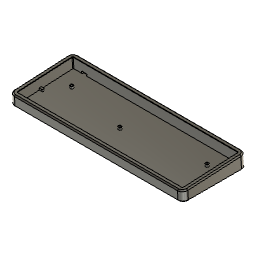
MFR60 (Autodesk Fusion 360 design; units mm, degrees)
Autodesk Fusion 360 part; units mm, degrees
note: some values were not read from the file. Set by a fixed rule: which sketch regions a step uses.
sketch "PCB Plane" plane through (0, 0, 0) normal (0, 0, 1) x (1, 0, 0)
  line L0 (0, 0) -> (285.75, 0) construction
  line L1 (285.75, 0) -> (285.75, 95.25) construction
  line L2 (285.75, 95.25) -> (0, 95.25) construction
  line L3 (0, 95.25) -> (0, 0) construction
  line L4 (-0.5, -0.5) -> (286.25, -0.5)
  line L5 (286.25, -0.5) -> (286.25, 95.75)
  line L6 (286.25, 95.75) -> (-0.5, 95.75)
  line L7 (-0.5, 95.75) -> (-0.5, -0.5)
  line L8 (-7.5, 102.75) -> (-7.5, -7.5)
  line L9 (-7.5, -7.5) -> (293.25, -7.5)
  line L10 (293.25, -7.5) -> (293.25, 102.75)
  line L11 (293.25, 102.75) -> (-7.5, 102.75)
  dimension "d1" = 285.75
  dimension "d2" = 95.25
  dimension "d3" = 0.5
  dimension "d4" = 7.5
  constraint horizontal L0
  constraint vertical L1
  constraint horizontal L2
  constraint vertical L3
  constraint coincident L0.start L3.end
  measures "d1" distance of L0.start L0.end
  measures "d2" distance of L0.start L2.end
ref_plane "WorkPlane1" through (142.875, 47.625, -3.46) normal (0, 0, 1) x (1, 0, 0)
ref_plane "WorkPlane2" through (142.875, 47.625, 14.6) normal (0, 0, 1) x (1, 0, 0)
extrude "Extrude1" add sketch "PCB Plane" along normal up to surface (14.6 mm away) and the other way up to surface (3.46 mm away)
sketch "Angle Sketch" plane through (293.25, 0, 0) normal (1, 0, 0) x (0, 1, 0)
  line L0 (102.75, 14.6) -> (-7.5, 14.6)
  line L1 (-7.5, 14.6) -> (-7.5, -3.46)
  line L2 (-7.5, -3.46) -> (102.75, -3.46)
  line L3 (102.75, -3.46) -> (102.75, 14.6)
  line L4 (-7.5, 14.6) -> (-7.5, -3.6755)
  line L5 (-7.5, -3.6755) -> (92.363, -8.9091)
  line L6 (-7.5, -3.6755) -> (92.5, -3.6755) construction
  dimension "d11" = 18.2755
  dimension "d12" = 100
  dimension "d13" = 3
  constraint coincident L0.end L1.start
  constraint perpendicular L0 L4
  constraint horizontal L6
  measures "d11" distance of L0.end L4.end
  measures "d12" distance of L4.end L5.end
  measures "d13" angle of L5 L6
ref_plane "WorkPlane3" through (293.25, 42.4315, -6.2923) normal (0, -0.052336, -0.99863) x (0, 0.99863, -0.052336)
sketch "Interior Base Plane" plane through (0, 0, -3.46) normal (0, 0, -1) x (1, 0, 0)
  line L0 (286.25, -95.75) -> (-0.5, -95.75)
  line L1 (-0.5, -95.75) -> (-0.5, 0.5)
  line L2 (-0.5, 0.5) -> (286.25, 0.5)
  line L3 (286.25, 0.5) -> (286.25, -95.75)
  line L4 (-7.5, 7.5) -> (-7.5, -102.75)
  line L5 (-7.5, -102.75) -> (293.25, -102.75)
  line L6 (293.25, -102.75) -> (293.25, 7.5)
  line L7 (293.25, 7.5) -> (-7.5, 7.5)
  line L8 (-7.5, 7.5) -> (293.25, 7.5)
  line L9 (293.25, 7.5) -> (293.25, -102.75)
  line L10 (293.25, -102.75) -> (-7.5, -102.75)
  line L11 (-7.5, -102.75) -> (-7.5, 7.5)
  constraint horizontal L8
  constraint vertical L9
  constraint horizontal L10
  constraint vertical L11
  constraint coincident L5.end L6.start
  constraint coincident L4.start L7.end
extrude "Extrude2" add sketch "Interior Base Plane" along normal up to surface contours L0 L1 L2 L3 | L4 L5 L6 L7 L8 L9 L10 L11 end surface through (293.25, 42.4315, -6.2923) normal (0, -0.052336, -0.99863) offset 0
fillet "Fillet1" radius 9 1 edges at (293.25, -7.5, 5.4623)
fillet "Fillet2" radius 9 1 edges at (293.25, 102.75, 2.5733)
fillet "Fillet3" radius 9 1 edges at (-7.5, 102.75, 2.5733)
fillet "Fillet4" radius 9 1 edges at (-7.5, -7.5, 5.4623)
fillet "Fillet5" radius 1 1 edges at (286.25, 95.75, 5.57)
fillet "Fillet6" radius 1 1 edges at (-0.5, 95.75, 5.57)
fillet "Fillet7" radius 1 1 edges at (286.25, -0.5, 5.57)
fillet "Fillet8" radius 1 1 edges at (-0.5, -0.5, 5.57)
chamfer "Chamfer1" distance 2 angle 45 8 edges at (-7.5, 47.625, 14.6) (-4.864, 100.114, 14.6) (142.875, 102.75, 14.6) (290.614, 100.114, 14.6) (293.25, 47.625, 14.6) (290.614, -4.864, 14.6) (142.875, -7.5, 14.6) (-4.864, -4.864, 14.6)
chamfer "Chamfer2" distance 2 angle 45 8 edges at (-7.5, 47.625, -6.5645) (-4.864, -4.864, -3.8136) (142.875, -7.5, -3.6755) (290.614, -4.864, -3.8136) (293.25, 47.625, -6.5645) (290.614, 100.114, -9.3153) (142.875, 102.75, -9.4535) (-4.864, 100.114, -9.3153)
chamfer "Chamfer3" distance 0.5 angle 45 4 edges at (142.875, 95.75, 14.6) (-0.5, 47.625, 14.6) (142.875, -0.5, 14.6) (286.25, 47.625, 14.6)
extrude "Extrude3" add 1 faces at (190, 65.3342, -7.4926) along direction (0, 0.052336, 0.99863) blind 1
ref_plane "WorkPlane4" through (142.875, 47.625, 0) normal (0, 0, 1) x (1, 0, 0)
sketch "USB C Hole Internal" plane through (0, 95.75, 0) normal (0, -1, 0) x (1, 0, 0)
  line L0 (285.25, 14.1) -> (0.5, 14.1)
  line L1 (0.5, -3.46) -> (285.25, -3.46)
  line L2 (15.4, -3.46) -> (21.75, -3.46)
  line L3 (23.3, -1.91) -> (23.3, -1.35)
  line L4 (21.75, 0.2) -> (15.4, 0.2)
  line L5 (13.85, -1.35) -> (13.85, -1.91)
  arc A0 (15.4, 0.2) -> (13.85, -1.35) centre (15.4, -1.35) ccw
  arc A1 (23.3, -1.35) -> (21.75, 0.2) centre (21.75, -1.35) ccw
  arc A2 (21.75, -3.46) -> (23.3, -1.91) centre (21.75, -1.91) ccw
  arc A3 (13.85, -1.91) -> (15.4, -3.46) centre (15.4, -1.91) ccw
  line L6 (0.5, 14.1) -> (0.5, -3.46)
  line L7 (285.25, -3.46) -> (285.25, 14.1)
  line L8 (285.25, -0.2545) -> (285.75, -0.2545)
  line L9 (18.575, 0.2) -> (18.575, -3.46) construction
  line L10 (285.75, -0.2545) -> (285.375, -0.2545)
  dimension "d36" = 1.55
  dimension "d82" = 0.5
  dimension "d83" = 4.725
  dimension "d89" = 3.66
  dimension "d90" = 3.66
  dimension "d132" = 0.375
  dimension "d133" = 266.8
  constraint horizontal L2
  constraint vertical L3
  constraint horizontal L4
  constraint vertical L5
  constraint tangent L5 A0
  constraint tangent L4 A0
  constraint tangent L4 A1
  constraint tangent L3 A1
  constraint equal A0 A1
  constraint tangent L2 A2
  constraint tangent L3 A2
  constraint equal A0 A2
  constraint tangent L2 A3
  constraint tangent L5 A3
  constraint equal A0 A3
  constraint coincident L7 L8.start
  constraint perpendicular L7 L8
  constraint midpoint L4 L9.start
  constraint midpoint L2 L9.end
  constraint perpendicular L7 L10
  measures "d36" radius of A0
  measures "d82" distance of L8.start L8.end
  measures "d83" distance of L5 L9
  measures "d89" distance of L2 L4
  measures "d90" distance of L1 L4
  measures "d132" distance of L8.end L10.end
  measures "d133" distance of L9 L10.end
extrude "Extrude4" cut sketch "USB C Hole Internal" against normal through all contours L1 L2 L3 L4 L5 A0 A1 A2 A3
sketch "USB C Hole External" plane through (0, 102.75, 0) normal (0, 1, 0) x (-1, 0, 0)
  line L0 (-21.75, 0.2) -> (-15.4, 0.2)
  arc A0 (-13.85, -1.35) -> (-15.4, 0.2) centre (-15.4, -1.35) ccw
  line L1 (-13.85, -1.35) -> (-13.85, -1.91)
  arc A1 (-15.4, -3.46) -> (-13.85, -1.91) centre (-15.4, -1.91) ccw
  line L2 (-15.4, -3.46) -> (-21.75, -3.46)
  arc A2 (-23.3, -1.91) -> (-21.75, -3.46) centre (-21.75, -1.91) ccw
  line L3 (-23.3, -1.91) -> (-23.3, -1.35)
  arc A3 (-21.75, 0.2) -> (-23.3, -1.35) centre (-21.75, -1.35) ccw
  line L4 (-284.25, -7.4535) -> (-1.5, -7.4535)
  line L5 (-1.5, -7.4535) -> (-1.5, 12.6)
  line L6 (-1.5, 12.6) -> (-284.25, 12.6)
  line L7 (-284.25, 12.6) -> (-284.25, -7.4535)
  line L8 (-13.85, -1.63) -> (-23.3, -1.63) construction
  line L9 (-18.575, 0.2) -> (-18.575, -3.46) construction
  line L10 (-19.075, 2.45) -> (-19.075, -5.71) construction
  line L11 (-190.8318, -1.63) -> (-176.8818, -1.63) construction
  line L12 (-21.75, 2.45) -> (-15.4, 2.45)
  line L13 (-11.6, -1.35) -> (-11.6, -1.91)
  line L14 (-15.4, -5.71) -> (-21.75, -5.71)
  line L15 (-25.55, -1.91) -> (-25.55, -1.35)
  arc A4 (-25.55, -1.91) -> (-21.75, -5.71) centre (-21.75, -1.91) ccw
  arc A5 (-21.75, 2.45) -> (-25.55, -1.35) centre (-21.75, -1.35) ccw
  arc A6 (-11.6, -1.35) -> (-15.4, 2.45) centre (-15.4, -1.35) ccw
  arc A7 (-15.4, -5.71) -> (-11.6, -1.91) centre (-15.4, -1.91) ccw
  dimension "d39" = 8.16
  dimension "d40" = 4.08
  dimension "d42" = 13.95
  dimension "d43" = 3.8
  dimension "d85" = 13.95
  dimension "d86" = 8.16
  dimension "d87" = 6.975
  dimension "d88" = 4.08
  constraint midpoint L1 L8.start
  constraint midpoint L3 L8.end
  constraint midpoint L0 L9.start
  constraint midpoint L2 L9.end
  constraint perpendicular L2 L10
  constraint perpendicular L10 L11
  constraint horizontal L12
  constraint vertical L13
  constraint horizontal L14
  constraint vertical L15
  constraint tangent L14 A4
  constraint tangent L15 A4
  constraint tangent L15 A5
  constraint tangent L12 A5
  constraint equal A4 A5
  constraint tangent L12 A6
  constraint tangent L13 A6
  constraint equal A4 A6
  constraint tangent L13 A7
  constraint tangent L14 A7
  constraint equal A4 A7
  measures "d39" distance of L10.start L10.end
  measures "d40" distance of L8 L10.start
  measures "d42" distance of L11.start L11.end
  measures "d43" radius of A4
  measures "d85" distance of L13 L15
  measures "d86" distance of L12 L14
  measures "d87" distance of L9 L15
  measures "d88" distance of L8.end L14
extrude "Extrude5" cut sketch "USB C Hole External" against normal blind 4.5025 contours L12 L13 L14 L15 A4 A5 A6 A7
chamfer "Chamfer4" distance 0.25 angle 45 8 edges at (24.437, 102.75, -4.597) (25.55, 102.75, -1.63) (24.437, 102.75, 1.337) (18.575, 102.75, 2.45) (12.713, 102.75, 1.337) (11.6, 102.75, -1.63) (12.713, 102.75, -4.597) (18.575, 102.75, -5.71)
sketch "Hole Tops" plane through (0, 0, 0) normal (0, 0, 1) x (1, 0, 0)
  line L0 (0, 0) -> (195.2625, 0) construction
  line L1 (195.2625, 0) -> (195.2625, 76.2) construction
  line L2 (195.2625, 76.2) -> (0, 76.2) construction
  line L3 (0, 76.2) -> (0, 0) construction
  line L4 (195.2625, 76.2) -> (195.2625, 57.15) construction
  line L5 (195.2625, 57.15) -> (193.1449, 57.15) construction
  circle A0 centre (157.1625, 57.15) radius 2.75
  circle A1 centre (38.1, 57.15) radius 2.75
  circle A2 centre (38.1, 19.05) radius 2.75
  circle A3 centre (157.1625, 19.05) radius 2.75
  dimension "d47" = 195.2625
  dimension "d48" = 76.2
  dimension "d51" = 19.05
  dimension "d52" = 38.1
  dimension "d53" = 19.05
  dimension "d54" = 38.1
  dimension "d55" = 38.1
  dimension "d56" = 19.05
  dimension "d57" = 38.1
  dimension "d58" = 19.05
  dimension "d59" = 5.5
  constraint horizontal L0
  constraint vertical L1
  constraint horizontal L2
  constraint vertical L3
  constraint coincident L0.start L3.end
  constraint perpendicular L2 L4
  constraint perpendicular L1 L5
  constraint equal A0 A1
  constraint equal A0 A3
  constraint equal A1 A2
  measures "d47" distance of L0.start L0.end
  measures "d48" distance of L0.start L2.end
  measures "d51" distance of L2 A0.centre
  measures "d52" distance of L1 A0.centre
  measures "d53" distance of L0 A3.centre
  measures "d54" distance of L1 A3.centre
  measures "d55" distance of L3 A2.centre
  measures "d56" distance of L0 A2.centre
  measures "d57" distance of L3 A1.centre
  measures "d58" distance of L2 A1.centre
  measures "d59" diameter of A1
sketch "Screwpost Positions" plane through (0, 0, -3.46) normal (0, 0, 1) x (-1, 0, 0)
  line L0 (0.5, -7.4953) -> (-286.25, -7.4953)
  line L1 (-286.25, -7.4953) -> (-286.25, -94.75)
  line L2 (-15.4, -95.75) -> (-0.5, -95.75)
  line L3 (0.5, -94.75) -> (0.5, -7.4953)
  line L4 (-21.75, -98.2475) -> (-15.4, -98.2475)
  line L5 (-15.4, -98.2475) -> (-15.4, -95.75)
  arc A0 (-0.5, -95.75) -> (0.5, -94.75) centre (-0.5, -94.75) ccw
  arc A1 (-286.25, -94.75) -> (-285.25, -95.75) centre (-285.25, -94.75) ccw
  line L6 (-285.25, -95.75) -> (-21.75, -95.75)
  line L7 (-21.75, -95.75) -> (-21.75, -98.2475)
  line L8 (0.5, -95.7494) -> (0, -95.7494) construction
  line L9 (0, -95.7494) -> (0, -95.2494) construction
  line L10 (0, -95.2494) -> (0.5, -95.2494) construction
  line L11 (0.5, -95.2494) -> (0.5, -95.7494) construction
  line L12 (0, -95.2494) -> (-285.75, -95.2494) construction
  line L13 (-285.75, -95.2494) -> (-285.75, 0.0006) construction
  line L14 (-285.75, 0.0006) -> (0, 0.0006) construction
  line L15 (0, 0.0006) -> (0, -95.2494) construction
  line L16 (0, -94.9244) -> (-285.75, -94.9244) construction
  line L17 (-285.75, -0.3244) -> (0, -0.3244) construction
  line L18 (-0.375, 0.0006) -> (-0.375, -95.2494) construction
  line L19 (-285.375, -95.2494) -> (-285.375, 0.0006) construction
  circle A2 centre (-25.575, -67.0244) radius 2.75
  circle A3 centre (-128.375, -47.9244) radius 2.75
  circle A4 centre (-190.875, -9.7244) radius 2.75
  circle A5 centre (-260.425, -67.0244) radius 2.75
  circle A6 centre (-3.875, -38.4244) radius 1.7
  line L20 (-3.875, -40.1244) -> (-0.375, -40.1244)
  line L21 (-3.875, -36.7244) -> (-0.375, -36.7244)
  line L22 (-0.375, -40.1244) -> (0.5, -40.1244)
  line L23 (-0.375, -36.7244) -> (0.5, -36.7244)
  circle A7 centre (-281.875, -38.4244) radius 1.7
  line L24 (-282.1379, -40.104) -> (-286.25, -40.104)
  line L25 (-281.875, -36.7244) -> (-286.25, -36.7244)
  line L26 (-3.875, -38.4244) -> (-281.875, -38.4244) construction
  line L27 (-3.875, -38.4244) -> (-5.375, -38.4244) construction
  line L28 (-281.875, -38.4244) -> (-280.375, -38.4244) construction
  line L29 (-21.75, -95.75) -> (-15.4, -95.75) construction
  line L30 (-18.575, -94.9244) -> (-18.575, -96.9244)
  dimension "d91" = 0.5
  dimension "d92" = 0.5
  dimension "d93" = 285.75
  dimension "d94" = 95.25
  dimension "d95" = 0.325
  dimension "d96" = 0.325
  dimension "d97" = 0.375
  dimension "d98" = 0.375
  dimension "d99" = 25.2
  dimension "d100" = 27.9
  dimension "d101" = 128
  dimension "d102" = 47
  dimension "d103" = 190.5
  dimension "d104" = 85.2
  dimension "d105" = 5.5
  dimension "d106" = 24.95
  dimension "d107" = 27.9
  dimension "d110" = 3.4
  dimension "d111" = 56.5
  dimension "d114" = 3.4
  dimension "d128" = 1.5
  dimension "d129" = 5
  dimension "d130" = 1.5
  dimension "d131" = 5
  dimension "d141" = 2
  constraint horizontal L8
  constraint vertical L9
  constraint horizontal L10
  constraint vertical L11
  constraint horizontal L12
  constraint vertical L13
  constraint horizontal L14
  constraint vertical L15
  constraint equal A2 A3
  constraint equal A2 A4
  constraint equal A2 A5
  constraint coincident A6 L20.start
  constraint coincident L18 L20.end
  constraint tangent A6 L20
  constraint perpendicular L18 L20
  constraint coincident A6 L21.start
  constraint coincident L18 L21.end
  constraint tangent A6 L21
  constraint perpendicular L18 L21
  constraint coincident L3 L22.end
  constraint perpendicular L3 L22
  constraint coincident L3 L23.end
  constraint perpendicular L3 L23
  constraint coincident A7 L24.start
  constraint coincident L1 L24.end
  constraint perpendicular L1 L24
  constraint coincident A7 L25.start
  constraint coincident L1 L25.end
  constraint tangent A7 L25
  constraint perpendicular L1 L25
  constraint coincident A6.centre L26.start
  constraint coincident A7.centre L26.end
  constraint parallel L12 L26
  constraint parallel L26 L27
  constraint parallel L26 L28
  constraint coincident L6.end L7.start
  constraint coincident L2.start L5.end
  constraint coincident L16 L30.start
  constraint perpendicular L29 L30
  measures "d91" distance of L8.start L8.end
  measures "d92" distance of L8.start L10.end
  measures "d93" distance of L9.end L12.end
  measures "d94" distance of L9.end L14.end
  measures "d99" distance of L18 A2.centre
  measures "d100" distance of L16 A2.centre
  measures "d101" distance of L18 A3.centre
  measures "d102" distance of L16 A3.centre
  measures "d103" distance of L18 A4.centre
  measures "d104" distance of L16 A4.centre
  measures "d105" diameter of A2
  measures "d106" distance of L19 A5.centre
  measures "d107" distance of L16 A5.centre
  measures "d110" diameter of A6
  measures "d111" distance of L16 A6.centre
  measures "d114" diameter of A7
  measures "d128" distance of A6.centre L27.end
  measures "d129" distance of L18 L27.end
  measures "d130" distance of A7.centre L28.end
  measures "d131" distance of L19 L28.end
  measures "d141" distance of L30.start L30.end
extrude "Extrude7" add sketch "Screwpost Positions" along normal blind 3.46 contours L0 A4 | L0 A4 | L3 A6 L20 L21 L22 L23 | A6 | L1 A7 L24 L25 | A7 | A2 | A3 | A5
hole "Hole5" at (260.425, 67.0244, 0) direction (0, 0, -1) diameter 3.2 depth 4 tip angle 180
hole "Hole6" at (128.375, 47.9244, 0) direction (0, 0, -1) diameter 3.2 depth 4 tip angle 180
hole "Hole7" at (190.875, 9.7244, 0) direction (0, 0, -1) diameter 3.2 depth 4 tip angle 180
hole "Hole8" at (25.575, 67.0244, 0) direction (0, 0, -1) diameter 3.2 depth 4 tip angle 180
move_body "Move1" bodies 1 to x (1, 0, 0) y (0, 0.99863, 0.052336) z (0, -0.052336, 0.99863) at (0, -0.2054, 0.2828)
equation "d87 = ( 13.95 / 2 ) * 1 mm"
equation "d88 = ( 8.16 / 2 ) * 1 mm"
equation "d93 = ( 15 * 19.05 ) * 1 mm"
equation "d94 = ( 5 * 19.05 ) * 1 mm"
